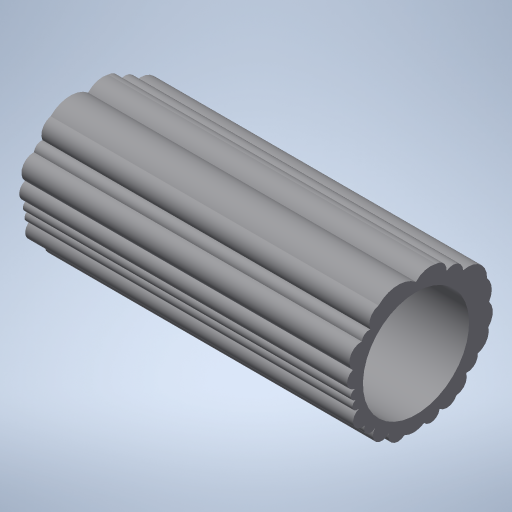
# Autodesk Inventor part: MANGA PAT1
Saved by Autodesk Inventor 2023 (Build 270158000, 158)
## iProperties
Created: 2022-10-06
Part Number: MANGA PAT1
Material: Generic
Document SubType Name: Modeling
Designer: Xiaba
Density: 1 g/cm^3
Appearance: Default
Author: Xiaba
Autodesk Inventor part; units mm, degrees
ref_plane "YZ Plane" through (0, 0, 0) normal (1, 0, 0) x (0, 1, 0)
ref_plane "XZ Plane" through (0, 0, 0) normal (0, 1, 0) x (-1, 0, 0)
ref_plane "XY Plane" through (0, 0, 0) normal (0, 0, 1) x (1, 0, 0)
sketch "Sketch1" plane through (0, 0, 0) normal (1, 0, 0) x (0, 1, 0)
  arc A0 (4.1909, 15.4186) -> (-0.0548, 14.932) centre (2.1329, 14.6094) ccw
  arc A1 (9.1315, 13.2306) -> (4.1909, 15.4186) centre (6.2427, 13.3796) ccw
  arc A2 (10.6369, 11.137) -> (9.1315, 13.2306) centre (8.8854, 11.4656) ccw
  arc A3 (14.6936, 9.1528) -> (10.6369, 11.137) centre (11.8437, 8.4653) ccw
  arc A4 (13.6712, -7.4537) -> (16.4772, -4.8768) centre (13.8806, -4.8655) ccw
  arc A5 (11.7816, -11.5139) -> (13.6712, -7.4537) centre (11.6995, -9.0059) ccw
  arc A6 (7.209, -17.333) -> (11.7816, -11.5139) centre (7.3993, -12.7763) ccw
  arc A7 (1.9798, -17.8261) -> (7.209, -17.333) centre (4.2694, -14.1335) ccw
  arc A8 (-3.2846, -17.6562) -> (1.9798, -17.8261) centre (-0.556, -14.7538) ccw
  arc A9 (-7.555, -15.0817) -> (-3.2846, -17.6562) centre (-4.102, -14.183) ccw
  arc A10 (-10.2552, -12.2375) -> (-7.555, -15.0817) centre (-7.7524, -12.5652) ccw
  arc A11 (-13.7925, -9.8762) -> (-10.2552, -12.2375) centre (-11.1236, -9.7082) ccw
  arc A12 (-14.6021, -5.7609) -> (-13.7925, -9.8762) centre (-12.703, -7.5246) ccw
  arc A13 (-15.7039, -1.9761) -> (-14.6021, -5.7609) centre (-14.3126, -3.6239) ccw
  arc A14 (-15.8788, 2.8495) -> (-15.7039, -1.9761) centre (-11.689, 0.5854) ccw
  arc A15 (-13.5313, 6.6942) -> (-15.8788, 2.8495) centre (-14.0938, 4.3987) ccw
  arc A16 (-10.712, 9.9696) -> (-13.5313, 6.6942) centre (-12.1638, 8.3682) ccw
  arc A17 (-9.0105, 12.5284) -> (-10.712, 9.9696) centre (-9.6928, 11.137) ccw
  arc A18 (-4.7007, 13.8984) -> (-9.0105, 12.5284) centre (-6.8182, 13.0957) ccw
  arc A19 (-2.4666, 14.7885) -> (-4.7007, 13.8984) centre (-3.5761, 14.3246) ccw
  arc A20 (-0.0548, 14.932) -> (-2.4666, 14.7885) centre (-1.2518, 14.7111) ccw
  arc A21 (15.1118, 0.025) -> (14.6936, 9.1528) centre (9.8039, 4.3553) ccw
  arc A22 (16.4772, -4.8768) -> (15.1118, 0.025) centre (11.7652, -3.5483) ccw
  point P0 (0, 0)
  point P1 (-10.7372, 9.9921)
  constraints: 50 point on circle, 23 centre point, 1 tangent
extrude "Extrusion1" add sketch "Sketch1" against normal blind 80
sketch "Sketch2" plane through (0, 0, 0) normal (1, 0, 0) x (0, 1, 0)
  circle A0 centre (0, 0) radius 12.953
  constraints: 1 centre point, 1 coincident
extrude "Extrusion2" cut sketch "Sketch2" against normal blind 81
body "Solid1"
